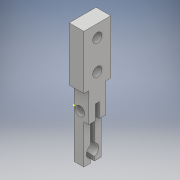
# Autodesk Inventor part: ferrule holder
Saved by Autodesk Inventor 2017 (Build 210142000, 142)
## iProperties
Created: 2018-04-15
Part Number: ferrule holder
Material: Generic
Document SubType Name: Modeling
Designer: dasae
Density: 1 g/cm^3
Appearance: Default
Author: dasae
Autodesk Inventor part; units mm, degrees
ref_plane "YZ Plane" through (0, 0, 0) normal (1, 0, 0) x (0, 1, 0)
ref_plane "XZ Plane" through (0, 0, 0) normal (0, 1, 0) x (-1, 0, 0)
ref_plane "XY Plane" through (0, 0, 0) normal (0, 0, 1) x (1, 0, 0)
sketch "Sketch2" plane through (0, 0, 0) normal (0, 1, 0) x (-1, 0, 0)
  line L0 (0, 0) -> (0, -10)
  line L1 (0, 0) -> (0, 10)
  line L2 (0, -10) -> (-2, -10)
  line L3 (-2, -10) -> (-2, -2)
  line L4 (-3, -2) -> (-2, -2)
  line L5 (-3, -2) -> (-3, -0.5) construction
  line L6 (-2, 10) -> (0, 10)
  line L7 (-3, -0.5) -> (0, -0.5) construction
  circle A0 centre (-1.2, -0.5) radius 0.95
  line L8 (-3, -2) -> (-3, 10)
  line L9 (-3, 10) -> (-2, 10)
  dimension "d0" = 10
  dimension "d1" = 10
  dimension "d2" = 2
  dimension "d9" = 1.9
  dimension "d10" = 8
  dimension "d11" = 3
  dimension "d12" = 1.8
  constraints: 20 end point, 4 perpendicular, 4 point on line, 2 horizontal, 2 vertical, 1 centre point
  measures "d0" distance of L0.start L0.end
  measures "d1" distance of L0.start L1.end
  measures "d2" distance of L0.end L2.end
  measures "d9" diameter of A0
  measures "d10" distance between parallel lines of L4 L2
  measures "d11" distance between parallel lines of L1 L8
  measures "d12" distance from line of L5 A0.centre
extrude "Extrusion1" add sketch "Sketch2" along normal blind 3.5
sketch "Sketch3" plane through (3, 0, 10) normal (1, 0, 0) x (0, 0, -1)
  line L0 (0, 0) -> (0, 3.5) projected
  line L1 (0, 1.75) -> (20, 1.75) construction
  line L2 (20, 1.75) -> (20, 2.15)
  line L3 (20, 0) -> (20, 3.5) projected
  line L4 (9, 2.15) -> (9, 1.35)
  line L5 (20, 2.15) -> (19.1843, 2.15)
  line L6 (16.8157, 2.15) -> (9, 2.15)
  line L7 (9, 1.35) -> (16.8157, 1.35)
  line L8 (19.1843, 1.35) -> (20, 1.35)
  arc A0 (16.8157, 1.35) -> (19.1843, 1.35) centre (18, 1.75) ccw
  arc A1 (19.1843, 2.15) -> (16.8157, 2.15) centre (18, 1.75) ccw
  line L9 (20, 1.75) -> (20, 1.35)
  point P0 (10, 0)
  dimension "d16" = 2
  dimension "d17" = 0.4
  dimension "d18" = 11
  dimension "d19" = 0.8
  constraints: 16 end point, 4 point on circle, 3 perpendicular, 3 point on line, 2 centre point, 1 horizontal, 1 midpoint, 1 vertical
  measures "d16" distance of A0.centre L1.end
  measures "d17" distance of L1.end L2.end
  measures "d18" distance of L2.end L4.start
  measures "d19" distance of L4.start L4.end
extrude "Extrusion2" cut sketch "Sketch3" against normal blind 10
sketch "Sketch4" plane through (0, 0, -10) normal (-1, 0, 0) x (0, 0, 1)
  point P0 (10, 0)
sketch "Sketch5" plane through (0, 0, -10) normal (-1, 0, 0) x (0, 0, 1)
  line L0 (11, 0) -> (14, 0)
  line L1 (8, 0) -> (20, 0) projected
  line L2 (14, 0) -> (14, -1)
  line L3 (14, -1) -> (20, -1)
  line L4 (20, 0) -> (14, 0)
  line L5 (14, 3.5) -> (14, 4.5)
  line L6 (14, 4.5) -> (20, 4.5)
  line L7 (20, 3.5) -> (14, 3.5)
  line L8 (20, 4.5) -> (25, 4.5)
  line L9 (25, 4.5) -> (25, -1)
  line L10 (25, -1) -> (20, -1)
  line L11 (20, 3.5) -> (20, 0)
  point P0 (10, 0)
  dimension "d22" = 3
  dimension "d23" = 1
  dimension "d24" = 1
  dimension "d27" = 5
  constraints: 22 end point, 4 perpendicular, 1 horizontal, 1 midpoint, 1 point on line, 1 vertical
  measures "d22" distance of L0.start L0.end
  measures "d23" distance of L0.end L2.end
  measures "d24" distance of L5.start L5.end
  measures "d27" distance of L6.end L8.end
extrude "Extrusion3" add sketch "Sketch5" against normal blind 3
sketch "Sketch6" plane through (0, 0, -10) normal (-1, 0, 0) x (0, 0, 1)
  line L0 (22, 1.75) -> (14, 1.75) construction
  line L1 (25, 4.5) -> (14, 4.5) projected
  circle A0 centre (22.5, 1.75) radius 0.95
  line L2 (25, -1) -> (25, 4.5) projected
  circle A1 centre (16.5, 1.75) radius 0.95
  point P0 (10, 0)
  dimension "d28" = 2.75
  dimension "d32" = 1.9
  dimension "d33" = 2.5
  dimension "d34" = 1.9
  dimension "d35" = 6
  constraints: 2 centre point, 2 end point, 2 point on line, 1 horizontal
  measures "d28" distance between parallel lines of L1 L0
  measures "d32" diameter of A0
  measures "d33" distance from line of L2 A0.centre
  measures "d34" diameter of A1
  measures "d35" distance of A1.centre A0.centre
extrude "Extrusion4" cut sketch "Sketch6" against normal blind 3
body "Solid1"
